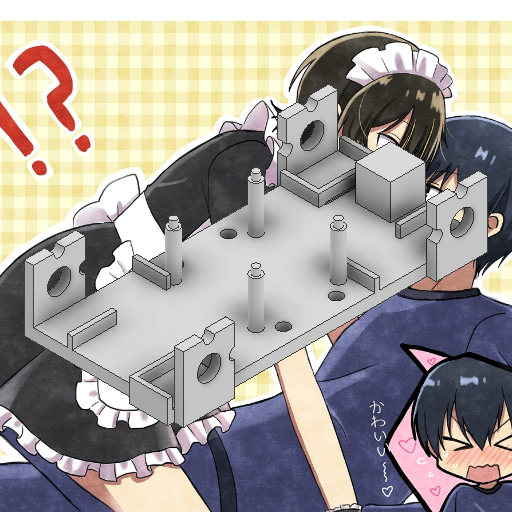
# Autodesk Inventor part: MainBody
Saved by Autodesk Inventor 2026.1 (Build 301233000, 233)
## iProperties
Created: 2026-05-04
Part Number: MainBody
Material: Generic
Document SubType Name: Modeling
Designer: 25adoh
Density: 1 g/cm^3
Appearance: Default
Author: 25adoh
Autodesk Inventor part; units mm, degrees
ref_plane "YZ Plane" through (0, 0, 0) normal (1, 0, 0) x (0, 1, 0)
ref_plane "XZ Plane" through (0, 0, 0) normal (0, 1, 0) x (-1, 0, 0)
ref_plane "XY Plane" through (0, 0, 0) normal (0, 0, 1) x (1, 0, 0)
sketch "Sketch1" plane through (0, 0, 0) normal (0, 1, 0) x (-1, 0, 0)
  line L0 (0, 0) -> (-60, 0)
  line L1 (-60, 0) -> (-60, -130)
  line L2 (-60, -130) -> (0, -130)
  line L3 (0, -130) -> (0, 0)
  line L4 (0, 0) -> (4, 0)
  line L5 (4, 0) -> (4, -22)
  line L6 (4, -22) -> (0, -22)
  line L7 (0, -22) -> (0, 0)
  line L8 (-60, 0) -> (-64, 0)
  line L9 (-64, 0) -> (-64, -22)
  line L10 (-64, -22) -> (-60, -22)
  line L11 (-60, -22) -> (-60, 0)
  line L12 (0, -130) -> (4, -130)
  line L13 (4, -130) -> (4, -108)
  line L14 (4, -108) -> (0, -108)
  line L15 (0, -108) -> (0, -130)
  line L16 (-60, -130) -> (-64, -130)
  line L17 (-64, -130) -> (-64, -108)
  line L18 (-64, -108) -> (-60, -108)
  line L19 (-60, -108) -> (-60, -130)
  circle A0 centre (-7, -53.7) radius 2.5
  circle A1 centre (-7, -76.3) radius 2.5
  circle A2 centre (-53, -53.7) radius 2.5
  circle A3 centre (-53, -76.3) radius 2.5
  line L20 (-45.5, -130) -> (-45.5, -111)
  line L21 (-45.5, -111) -> (-43.5, -111)
  line L22 (-43.5, -111) -> (-43.5, -130)
  line L23 (-14.5, 0) -> (-14.5, -19)
  line L24 (-14.5, -19) -> (-16.5, -19)
  line L25 (-16.5, -19) -> (-16.5, 0)
  line L26 (-16.5, 0) -> (-14.5, 0)
  line L27 (-16.5, -130) -> (-14.5, -130)
  line L28 (-45.5, -130) -> (-43.5, -130)
  circle A4 centre (-12.4, -47.4) radius 1.5
  circle A5 centre (-12.4, -82.6) radius 1.5
  circle A6 centre (-47.6, -47.4) radius 1.5
  circle A7 centre (-47.6, -82.6) radius 1.5
  circle A8 centre (-47.6, -82.6) radius 2.5
  circle A9 centre (-47.6, -47.4) radius 2.5
  circle A10 centre (-12.4, -47.4) radius 2.5
  circle A11 centre (-12.4, -82.6) radius 2.5
  line L29 (-46, -87.8) -> (-60, -87.8)
  line L30 (-46, -87.8) -> (-46, -85.8)
  line L31 (-46, -85.8) -> (-60, -85.8)
  line L32 (0, 0) -> (-14.5, 0)
  line L33 (-14.5, -42.2) -> (0, -42.2)
  line L34 (-14.5, -42.2) -> (-14.5, -44.2)
  line L35 (-14.5, -44.2) -> (0, -44.2)
  line L36 (-43.5, 0) -> (-43.5, -22.75)
  line L37 (-45.5, 0) -> (-45.5, -22.75)
  line L38 (-45.5, -22.75) -> (-43.5, -22.75)
  line L39 (-43.5, -22.75) -> (-43.5, -24.75)
  line L40 (-43.5, 0) -> (-45.5, 0)
  line L41 (-43.5, -24.75) -> (-60, -24.75)
  line L42 (-45.5, -22.75) -> (-60, -22.75)
  line L43 (-14.5, -130) -> (-14.5, -107.25)
  line L44 (-14.5, -107.25) -> (0, -107.25)
  line L45 (-16.5, -130) -> (-16.5, -107.25)
  line L46 (-16.5, -107.25) -> (-14.5, -107.25)
  line L47 (-16.5, -107.25) -> (-16.5, -105.25)
  line L48 (-16.5, -105.25) -> (0, -105.25)
  line L49 (-45.5, 0) -> (-45.5, 0.6)
  line L50 (-60, 0) -> (-60, 0.6)
  line L51 (-60, 0.6) -> (-45.5, 0.6)
  line L52 (-60, 0.6) -> (-60, 2.6)
  line L53 (-60, 2.6) -> (-43.5, 2.6)
  line L54 (-43.5, 2.6) -> (-43.5, 0)
  line L55 (-16.5, -130) -> (-16.5, -130.6)
  line L56 (-16.5, -130.6) -> (0, -130.6)
  line L57 (-16.5, -130.6) -> (-16.5, -132.6)
  line L58 (-16.5, -132.6) -> (0, -132.6)
  line L59 (0, -132.6) -> (0, -130.6)
  line L60 (0, -130.6) -> (0, -130)
  line L61 (-45.5, -130.6) -> (-45.5, -66.7979)
  line L62 (-14.5, -130) -> (-14.5, -130.6)
  point P0 (-30, -65)
  dimension "d0" = 60
  dimension "d1" = 130
  dimension "d2" = 4
  dimension "d3" = 22
  dimension "d4" = 4
  dimension "d5" = 22
  dimension "d6" = 4
  dimension "d7" = 22
  dimension "d8" = 4
  dimension "d9" = 22
  dimension "d52" = 5
  dimension "d53" = 5
  dimension "d64" = 14.5
  dimension "d66" = 19
  dimension "d67" = 2
  dimension "d74" = 19
  dimension "d75" = 2
  dimension "d84" = 3
  dimension "d86" = 3
  dimension "d88" = 3
  dimension "d90" = 3
  dimension "d91" = 5
  dimension "d92" = 5
  dimension "d93" = 5
  dimension "d94" = 5
  dimension "d100" = 2
  dimension "d102" = 2
  dimension "d107" = 22.75
  dimension "d108" = 2
  dimension "d109" = 22.75
  dimension "d110" = 2
  dimension "d111" = 0.6
  dimension "d112" = 2
  dimension "d113" = 0.6
  dimension "d114" = 2
  constraints: 126 end point, 27 perpendicular, 19 point on line, 12 centre point, 12 parallel, 10 vertical, 7 horizontal, 4 coincident, 4 collinear
  measures "d0" distance of L2.end L1.end
  measures "d1" distance of L1.end L0.end
  measures "d2" distance of L5.end L6.end
  measures "d3" distance of L4.end L5.end
  measures "d4" distance of L10.end L9.end
  measures "d5" distance of L9.end L8.end
  measures "d6" distance of L14.end L13.end
  measures "d7" distance of L13.end L12.end
  measures "d8" distance of L17.end L18.end
  measures "d9" distance of L16.end L17.end
  measures "d52" diameter of A2
  measures "d53" diameter of A3
  measures "d64" distance of L1.end L20.start
  measures "d66" distance of L20.start L20.end
  measures "d67" distance of L20.end L21.end
  measures "d74" distance of L23.start L23.end
  measures "d75" distance of L23.end L24.end
  measures "d84" diameter of A4
  measures "d86" diameter of A5
  measures "d88" diameter of A6
  measures "d90" diameter of A7
  measures "d91" diameter of A8
  measures "d92" diameter of A9
  measures "d93" diameter of A10
  measures "d94" diameter of A11
  measures "d100" distance of L29.start L30.end
  measures "d102" distance of L33.start L34.end
  measures "d107" distance of L36.start L36.end
  measures "d108" distance of L36.end L39.end
  measures "d109" distance of L27.end L43.end
  measures "d110" distance of L45.end L47.end
  measures "d111" distance of L37.start L49.end
  measures "d112" distance of L50.end L52.end
  measures "d113" distance of L27.start L55.end
  measures "d114" distance of L55.end L57.end
extrude "Extrusion1" add sketch "Sketch1" along normal blind 5 contours L3 L33 L34 L35 L48 L47 L45 L2 L22 L21 L20 L1 L29 L30 L31 L41 L39 L36 L0 L25 L24 L23 | L23 L24 L25 L0 | L3 L35 L34 L33 | L36 L38 L37 L0 | L0 L49 L51 L52 L53 L54 | L37 L42 L1 L0 | L0 L50 L51 L49 | L39 L41 L1 L42 L38 | L3 L44 L46 L47 L48 | L3 L2 L43 L44 | L43 L2 L45 L46 | L31 L30 L29 L1 | L60 L56 L62 L2 | L62 L56 L55 L2 | L59 L58 L57 L56 | L2 L20 L21 L22 | A4 | A5 | A6 | A7 | A8 L61 | L61 A8 | A9 | A10 | A11
extrude "Extrusion2" add sketch "Sketch1" along normal blind 28 contours L4 L5 L6 L3 | L1 L10 L9 L8 | L14 L13 L12 L3 | L1 L16 L17 L18
sketch "Sketch2" plane through (64, 0, 0) normal (1, 0, 0) x (0, 0, -1)
  line L0 (0, 28) -> (22, 28) projected
  line L1 (22, 0) -> (22, 28) projected
  line L2 (0, 28) -> (0, 5)
  line L3 (0, 5) -> (22, 5)
  line L4 (0, 28) -> (22, 5)
  line L5 (22, 0) -> (22, 28) projected
  line L6 (0, 5) -> (22, 28)
  circle A0 centre (11, 16.5) radius 5
  line L7 (108, 28) -> (130, 28)
  line L8 (108, 0) -> (108, 28)
  line L9 (130, 0) -> (130, 28)
  line L10 (108, 28) -> (108, 5)
  line L11 (108, 5) -> (130, 5)
  line L12 (108, 28) -> (130, 5)
  line L13 (130, 0) -> (130, 28)
  line L14 (108, 5) -> (130, 28)
  circle A1 centre (119, 16.5) radius 5
  line L15 (108, 28) -> (130, 28) projected
  line L16 (108, 0) -> (108, 28) projected
  line L17 (130, 0) -> (130, 28) projected
  line L18 (0, 28) -> (0, 5)
  line L19 (11, 28) -> (11.25, 28) construction
  circle A2 centre (11, 27.75) radius 2.25
  circle A3 centre (119, 27.75) radius 2.25
  circle A4 centre (22, 16.5) radius 2.5
  circle A5 centre (108, 16.5) radius 2.5
  dimension "d14" = 23
  dimension "d15" = 10
  dimension "d16" = 23
  dimension "d17" = 10
  dimension "d60" = 4.5
  dimension "d61" = 4.5
  dimension "d115" = 5
  dimension "d116" = 5
  constraints: 28 end point, 6 centre point, 5 point on line, 3 midpoint, 3 perpendicular, 2 coincident, 1 horizontal
  measures "d14" distance of L0.start L2.end
  measures "d15" diameter of A0
  measures "d16" distance of L7.start L10.end
  measures "d17" diameter of A1
  measures "d60" diameter of A2
  measures "d61" diameter of A3
  measures "d115" diameter of A4
  measures "d116" diameter of A5
extrude "Extrusion3" cut sketch "Sketch2" against normal blind 68 contours A2 L0 | L0 A2 | A0 L6 L4 | L4 L6 A0 | L6 L4 A0 | L6 A0 L4 | A4 L1 | L1 A4 | A3 L7 | L7 A3 | A5 L8 | L8 A5 | A1 L14 L12 | L12 L14 A1 | L14 A1 L12 | L12 A1 L14
sketch "Sketch3" plane through (0, 5, 0) normal (0, 1, 0) x (1, 0, 0)
  line L0 (60, 0) -> (43, 0)
  line L1 (-4, 0) -> (64, 0) projected
  line L2 (60, 22) -> (60, 0) projected
  line L3 (60, 22) -> (43, 22)
  line L4 (43, 22) -> (43, 0)
  line L5 (43, 0) -> (25, 0)
  line L6 (25, 0) -> (25, 22)
  line L7 (25, 22) -> (43, 22)
  line L8 (43, 7.25) -> (37.5, 7.25)
  line L9 (37.5, 7.25) -> (37.5, 14.75)
  line L10 (37.5, 14.75) -> (43, 14.75)
  line L11 (0, 130) -> (17, 130)
  line L12 (0, 108) -> (0, 130)
  line L13 (0, 108) -> (17, 108)
  line L14 (17, 108) -> (17, 130)
  line L15 (17, 130) -> (35, 130)
  line L16 (35, 130) -> (35, 108)
  line L17 (35, 108) -> (17, 108)
  line L18 (17, 122.75) -> (22.5, 122.75)
  line L19 (22.5, 122.75) -> (22.5, 115.25)
  line L20 (22.5, 115.25) -> (17, 115.25)
  line L21 (0, 108) -> (0, 130) projected
  line L22 (60, 130) -> (0, 130) projected
  point P0 (0, 0)
  point P1 (-4, 130)
  dimension "d20" = 17
  dimension "d21" = 18
  dimension "d24" = 7.5
  dimension "d25" = 5.5
  dimension "d26" = 17
  dimension "d27" = 18
  dimension "d28" = 7.5
  dimension "d29" = 5.5
  constraints: 38 end point, 10 perpendicular, 6 point on line, 2 horizontal
  measures "d20" distance of L0.start L0.end
  measures "d21" distance of L0.end L5.end
  measures "d24" distance of L8.end L9.end
  measures "d25" distance of L8.start L8.end
  measures "d26" distance of L11.start L11.end
  measures "d27" distance of L11.end L15.end
  measures "d28" distance of L18.end L19.end
  measures "d29" distance of L18.start L18.end
extrude "Extrusion4" add sketch "Sketch3" along normal blind 0.5 contours L0 L4 L3 L2 | L11 L14 L13 L12
sketch "Sketch4" plane through (0, 5, 0) normal (0, 1, 0) x (1, 0, 0)
  line L0 (60, 130) -> (17, 130) projected
  line L1 (17, 130) -> (0, 130) projected
  line L2 (0, 130) -> (-4, 130) projected
  line L3 (0, 130) -> (60, 130)
  line L4 (34, 130) -> (26, 130)
  line L5 (37.5, 130) -> (22.5, 130)
  line L6 (37.5, 130) -> (22.5, 130)
  line L7 (22.5, 130) -> (22.5, 115)
  line L8 (22.5, 115) -> (37.5, 115)
  line L9 (37.5, 115) -> (37.5, 130)
  line L10 (34, 130) -> (26, 130)
  line L11 (26, 130) -> (26, 124)
  line L12 (26, 124) -> (34, 124)
  line L13 (34, 124) -> (34, 130)
  point P0 (0, 0)
  point P1 (30, 130)
  dimension "d32" = 8
  dimension "d33" = 15
  dimension "d34" = 15
  dimension "d35" = 15
  dimension "d36" = 8
  dimension "d37" = 6
  constraints: 22 end point, 4 parallel, 3 midpoint, 2 horizontal, 2 perpendicular, 2 point on line, 1 collinear
  measures "d32" distance of L4.start L4.end
  measures "d33" distance of L5.start L5.end
  measures "d34" distance of L8.end L7.end
  measures "d35" distance of L7.end L6.end
  measures "d36" distance of L12.end L11.end
  measures "d37" distance of L11.end L10.end
extrude "Extrusion5" add sketch "Sketch4" along normal blind 15
sketch "Sketch5" plane through (64, 0, -130) normal (0, 0, -1) x (-1, 0, 0)
  line L0 (41.5, 5) -> (41.5, 20) projected
  line L1 (68, 0) -> (68, 28) projected
  line L2 (64, 28) -> (68, 28) projected
  line L3 (64, 5.5) -> (64, 28) projected
  line L4 (47, 5.5) -> (64, 5.5) projected
  line L5 (47, 5) -> (47, 5.5) projected
  line L6 (41.5, 5) -> (47, 5) projected
  line L7 (41.5, 5) -> (41.5, 20) projected
  line L8 (26.5, 20) -> (41.5, 20) projected
  line L9 (26.5, 5) -> (26.5, 20) projected
  line L10 (4, 5) -> (26.5, 5) projected
  line L11 (4, 5) -> (4, 28) projected
  line L12 (0, 28) -> (4, 28) projected
  line L13 (0, 0) -> (0, 28) projected
  line L14 (34, 20) -> (34, 5)
  line L15 (26.5, 5) -> (41.5, 5) projected
  line L16 (34, 5) -> (34, 13)
  line L17 (30, 13) -> (38, 13)
  line L18 (38, 13) -> (38, 5)
  line L19 (30, 13) -> (30, 5)
  line L20 (64, 0) -> (68, 0) projected
  line L21 (0, 0) -> (47.5, 0) projected
  line L22 (47.5, 0) -> (47.5, 5) projected
  line L23 (64, 5) -> (47.5, 5) projected
  line L24 (64, 0) -> (64, 5) projected
  dimension "d40" = 8
  dimension "d41" = 8
  constraints: 10 end point, 3 midpoint, 3 point on line, 2 perpendicular, 1 horizontal
  measures "d40" distance of L14.end L16.end
  measures "d41" distance of L17.start L17.end
extrude "Extrusion6" cut sketch "Sketch5" against normal blind 6 contours L15 L14 L17 L18 | L15 L19 L17 L14
extrude "Extrusion7" add sketch "Sketch1" along normal blind 10 contours L23 L24 L25 L0 | L3 L35 L34 L33 | L36 L38 L37 L0 | L0 L49 L51 L52 L53 L54 | L39 L41 L1 L42 L38 | L3 L44 L46 L47 L48 | L43 L2 L45 L46 | L31 L30 L29 L1 | L62 L56 L55 L2 | L59 L58 L57 L56 | L2 L20 L21 L22 | A4 | A5 | A6 | A7 | A8 L61 | L61 A8 | A9 | A10 | A11
extrude "Extrusion8" add sketch "Sketch1" along normal blind 25 contours A4 | A5 | A6 | A7 | A8 L61 | L61 A8 | A9 | A10 | A11
extrude "Extrusion9" add sketch "Sketch1" along normal blind 28 contours A4 | A5 | A6 | A7
body "Solid1"
